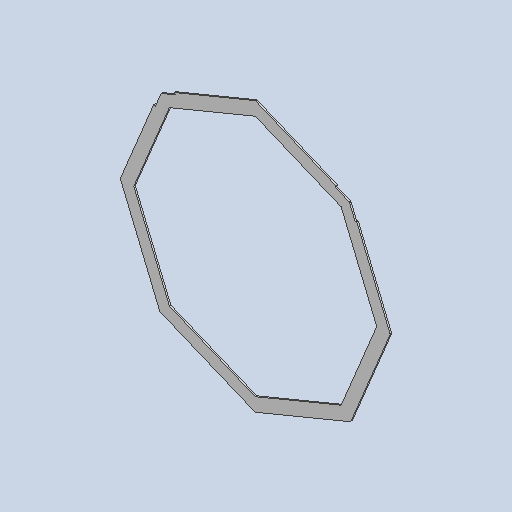
# Autodesk Inventor part: ДМС 104.1 Сектор кольца усилителя барабана полный
Saved by Autodesk Inventor 2024.2 (Build 282272000, 272)
## iProperties
Created: 2024-04-30
Part Number: ДМС 104.1 Сектор кольца усилителя барабана полный
Material: Generic
Document SubType Name: Sheet Metal
Designer: pokla
Density: 1 g/cm^3
Appearance: Default
Sheet Metal Rule: Default
Author: pokla
Autodesk Inventor part; units mm, degrees
ref_plane "YZ Plane" through (0, 0, 0) normal (1, 0, 0) x (0, 1, 0)
ref_plane "XZ Plane" through (0, 0, 0) normal (0, 1, 0) x (-1, 0, 0)
ref_plane "XY Plane" through (0, 0, 0) normal (0, 0, 1) x (1, 0, 0)
sketch "Sketch1" plane through (0, 0, 0) normal (0, 0, 1) x (1, 0, 0)
  line L0 (1.1481, 270.1225) -> (190.1937, 191.8173)
  line L1 (191.8173, 190.1937) -> (270.1225, 1.1481)
  line L2 (270.1225, -1.1481) -> (191.8173, -190.1937)
  line L3 (190.1937, -191.8173) -> (1.1481, -270.1225)
  line L4 (-1.1481, -270.1225) -> (-190.1937, -191.8173)
  line L5 (-191.8173, -190.1937) -> (-270.1225, -1.1481)
  line L6 (-270.1225, 1.1481) -> (-191.8173, 190.1937)
  line L7 (-190.1937, 191.8173) -> (-1.1481, 270.1225)
  line L8 (172.2075, 172.2075) -> (0, 243.5382)
  line L9 (0, 243.5382) -> (-172.2075, 172.2075)
  line L10 (-172.2075, 172.2075) -> (-243.5382, 0)
  line L11 (-243.5382, 0) -> (-172.2075, -172.2075)
  line L12 (-172.2075, -172.2075) -> (0, -243.5382)
  line L13 (0, -243.5382) -> (172.2075, -172.2075)
  line L14 (172.2075, -172.2075) -> (243.5382, 0)
  line L15 (243.5382, 0) -> (172.2075, 172.2075)
  arc A0 (1.1481, 270.1225) -> (-1.1481, 270.1225) centre (0, 267.3509) ccw
  arc A1 (-190.1937, 191.8173) -> (-191.8173, 190.1937) centre (-189.0456, 189.0456) ccw
  arc A2 (-270.1225, 1.1481) -> (-270.1225, -1.1481) centre (-267.3509, 0) ccw
  arc A3 (-191.8173, -190.1937) -> (-190.1937, -191.8173) centre (-189.0456, -189.0456) ccw
  arc A4 (-1.1481, -270.1225) -> (1.1481, -270.1225) centre (0, -267.3509) ccw
  arc A5 (190.1937, -191.8173) -> (191.8173, -190.1937) centre (189.0456, -189.0456) ccw
  arc A6 (270.1225, -1.1481) -> (270.1225, 1.1481) centre (267.3509, 0) ccw
  arc A7 (191.8173, 190.1937) -> (190.1937, 191.8173) centre (189.0456, 189.0456) ccw
  point P0 (0, 0)
  point P1 (0, 0)
  point P2 (0, 270.5981)
  point P3 (191.3417, 191.3417)
  point P4 (270.5981, 0)
  point P5 (191.3417, -191.3417)
  point P6 (0, -270.5981)
  point P7 (-191.3417, -191.3417)
  point P8 (-270.5981, 0)
  point P9 (-191.3417, 191.3417)
  dimension "d18" = 500
  dimension "d19" = 25
  dimension "d20" = 3
  dimension "d22" = 3
  measures "d18" distance between parallel lines of L2 L6
  measures "d19" distance between parallel lines of L0 L8
  measures "d20" radius of A0
  measures "d22" radius of A7
extrude "Plate2" add sketch "Sketch1" against normal blind 3
sketch "Sketch3" plane through (0, 0, 0) normal (0, 0, 1) x (1, 0, 0)
  line L0 (-191.8173, 190.1937) -> (-270.1225, 1.1481) projected
  arc A0 (-190.1937, 191.8173) -> (-191.8173, 190.1937) centre (-189.0456, 189.0456) ccw projected
  line L1 (-1.1481, 270.1225) -> (-190.1937, 191.8173) projected
  line L2 (-200.2363, 160.7224) -> (-189.1385, 187.5149)
  line L3 (-187.5149, 189.1385) -> (-160.7224, 200.2363)
  arc A1 (-187.5149, 189.1385) -> (-189.1385, 187.5149) centre (-186.3668, 186.3668) ccw
  line L4 (-162.0618, 203.4699) -> (-160.7224, 200.2363)
  line L5 (-200.2363, 160.7224) -> (-203.4699, 162.0618)
  point P0 (0, 0)
  dimension "d23" = 3.5
  dimension "d24" = 3
  dimension "d25" = 29
  dimension "d26" = 3.5
  constraints: 8 end point, 2 perpendicular, 2 point on circle, 2 point on line, 2 tangent, 1 centre point, 1 equal length, 1 parallel
  measures "d23" distance between parallel lines of L1 L3
  measures "d24" radius of A1
  measures "d25" distance of L3.end L3.start
  measures "d26" distance between parallel lines of L2 L0
extrude "Extrusion1" cut sketch "Sketch3" against normal up to surface (3 mm away)
mirror "Mirror1" about plane through (0, 0, 0) normal (1, 0, 0) of "Extrusion1"
equation "\"d22\" = d20"
equation "\"d21\" = Thickness"
equation "\"BendRadius\" = Thickness"
equation "\"BendReliefWidth\" = Thickness"
equation "\"BendReliefDepth\" = 0.5 * Thickness"
equation "\"CornerReliefSize\" = 4 * Thickness"
equation "\"MinimumRemnant\" = 2 * Thickness"
equation "\"TransitionRadius\" = BendRadius"
equation "\"JacobiRadiusSize\" = BendRadius"
equation "\"GapSize\" = Thickness"
equation "\"Thickness\" = 3"
body "Solid2"
